Autodesk Fusion 360 part; units mm, degrees
note: some values were not read from the file. Set by a fixed rule: which sketch regions a step uses.
(part 2 of 3)
  line L917 (15.6798, -39.6054) -> (15.6321, -39.5578)
  line L918 (15.2055, -47.9863) -> (15.2532, -47.8435)
  line L919 (15.2532, -47.8435) -> (15.3008, -47.7959)
  line L920 (15.3008, -47.7959) -> (15.396, -47.7482)
  line L921 (15.396, -47.7482) -> (15.5389, -47.7482)
  line L922 (15.5389, -47.7482) -> (15.6341, -47.7959)
  line L923 (15.6341, -47.7959) -> (15.6817, -47.8435)
  line L924 (15.6817, -47.8435) -> (15.7293, -47.9387)
  line L925 (15.7293, -47.9387) -> (15.7293, -48.3197)
  line L926 (15.7293, -48.3197) -> (14.7293, -48.3197)
  line L927 (14.7293, -48.3197) -> (14.7293, -47.9863)
  line L928 (14.7293, -47.9863) -> (14.777, -47.8911)
  line L929 (14.777, -47.8911) -> (14.8246, -47.8435)
  line L930 (14.8246, -47.8435) -> (14.9198, -47.7959)
  line L931 (14.9198, -47.7959) -> (15.0151, -47.7959)
  line L932 (15.0151, -47.7959) -> (15.1103, -47.8435)
  line L933 (15.1103, -47.8435) -> (15.1579, -47.8911)
  line L934 (15.1579, -47.8911) -> (15.2055, -47.9863)
  line L935 (15.2055, -47.9863) -> (15.2055, -48.3197)
  line L936 (14.7293, -47.3197) -> (15.5389, -47.3197)
  line L937 (15.5389, -47.3197) -> (15.6341, -47.2721)
  line L938 (15.6341, -47.2721) -> (15.6817, -47.2244)
  line L939 (15.6817, -47.2244) -> (15.7293, -47.1292)
  line L940 (15.7293, -47.1292) -> (15.7293, -46.9387)
  line L941 (15.7293, -46.9387) -> (15.6817, -46.8435)
  line L942 (15.6817, -46.8435) -> (15.6341, -46.7959)
  line L943 (15.6341, -46.7959) -> (15.5389, -46.7482)
  line L944 (15.5389, -46.7482) -> (14.7293, -46.7482)
  line L945 (14.7293, -46.4149) -> (14.7293, -45.8435)
  line L946 (15.7293, -46.1292) -> (14.7293, -46.1292)
  line L947 (14.7293, -45.653) -> (14.7293, -45.0816)
  line L948 (15.7293, -45.3673) -> (14.7293, -45.3673)
  line L949 (14.7293, -44.5578) -> (14.7293, -44.3673)
  line L950 (14.7293, -44.3673) -> (14.777, -44.2721)
  line L951 (14.777, -44.2721) -> (14.8722, -44.1768)
  line L952 (14.8722, -44.1768) -> (15.0627, -44.1292)
  line L953 (15.0627, -44.1292) -> (15.396, -44.1292)
  line L954 (15.396, -44.1292) -> (15.5865, -44.1768)
  line L955 (15.5865, -44.1768) -> (15.6817, -44.2721)
  line L956 (15.6817, -44.2721) -> (15.7293, -44.3673)
  line L957 (15.7293, -44.3673) -> (15.7293, -44.5578)
  line L958 (15.7293, -44.5578) -> (15.6817, -44.653)
  line L959 (15.6817, -44.653) -> (15.5865, -44.7482)
  line L960 (15.5865, -44.7482) -> (15.396, -44.7959)
  line L961 (15.396, -44.7959) -> (15.0627, -44.7959)
  line L962 (15.0627, -44.7959) -> (14.8722, -44.7482)
  line L963 (14.8722, -44.7482) -> (14.777, -44.653)
  line L964 (14.777, -44.653) -> (14.7293, -44.5578)
  line L965 (15.7293, -43.7006) -> (14.7293, -43.7006)
  line L966 (14.7293, -43.7006) -> (15.7293, -43.1292)
  line L967 (15.7293, -43.1292) -> (14.7293, -43.1292)
  line L968 (15.6817, -42.7006) -> (15.7293, -42.5578)
  line L969 (15.7293, -42.5578) -> (15.7293, -42.3197)
  line L970 (15.7293, -42.3197) -> (15.6817, -42.2244)
  line L971 (15.6817, -42.2244) -> (15.6341, -42.1768)
  line L972 (15.6341, -42.1768) -> (15.5389, -42.1292)
  line L973 (15.5389, -42.1292) -> (15.4436, -42.1292)
  line L974 (15.4436, -42.1292) -> (15.3484, -42.1768)
  line L975 (15.3484, -42.1768) -> (15.3008, -42.2244)
  line L976 (15.3008, -42.2244) -> (15.2532, -42.3197)
  line L977 (15.2532, -42.3197) -> (15.2055, -42.5102)
  line L978 (15.2055, -42.5102) -> (15.1579, -42.6054)
  line L979 (15.1579, -42.6054) -> (15.1103, -42.653)
  line L980 (15.1103, -42.653) -> (15.0151, -42.7006)
  line L981 (15.0151, -42.7006) -> (14.9198, -42.7006)
  line L982 (14.9198, -42.7006) -> (14.8246, -42.653)
  line L983 (14.8246, -42.653) -> (14.777, -42.6054)
  line L984 (14.777, -42.6054) -> (14.7293, -42.5102)
  line L985 (14.7293, -42.5102) -> (14.7293, -42.2721)
  line L986 (14.7293, -42.2721) -> (14.777, -42.1292)
  line L987 (34.3226, -25.4531) -> (34.3226, -26.2626)
  line L988 (34.3226, -26.2626) -> (34.3702, -26.3578)
  line L989 (34.3702, -26.3578) -> (34.4179, -26.4054)
  line L990 (34.4179, -26.4054) -> (34.5131, -26.4531)
  line L991 (34.5131, -26.4531) -> (34.7036, -26.4531)
  line L992 (34.7036, -26.4531) -> (34.7988, -26.4054)
  line L993 (34.7988, -26.4054) -> (34.8464, -26.3578)
  line L994 (34.8464, -26.3578) -> (34.894, -26.2626)
  line L995 (34.894, -26.2626) -> (34.894, -25.4531)
  line L996 (35.894, -26.4531) -> (35.3226, -26.4531)
  line L997 (35.6083, -26.4531) -> (35.6083, -25.4531)
  line L998 (35.6083, -25.4531) -> (35.5131, -25.5959)
  line L999 (35.5131, -25.5959) -> (35.4179, -25.6912)
  line L1000 (35.4179, -25.6912) -> (35.3226, -25.7388)
  line L1001 (38.9893, -52.5224) -> (39.1036, -52.5605)
  line L1002 (39.1036, -52.5605) -> (39.294, -52.5605)
  line L1003 (39.294, -52.5605) -> (39.3702, -52.5224)
  line L1004 (39.3702, -52.5224) -> (39.4083, -52.4844)
  line L1005 (39.4083, -52.4844) -> (39.4464, -52.4082)
  line L1006 (39.4464, -52.4082) -> (39.4464, -52.332)
  line L1007 (39.4464, -52.332) -> (39.4083, -52.2558)
  line L1008 (39.4083, -52.2558) -> (39.3702, -52.2177)
  line L1009 (39.3702, -52.2177) -> (39.294, -52.1796)
  line L1010 (39.294, -52.1796) -> (39.1417, -52.1415)
  line L1011 (39.1417, -52.1415) -> (39.0655, -52.1034)
  line L1012 (39.0655, -52.1034) -> (39.0274, -52.0653)
  line L1013 (39.0274, -52.0653) -> (38.9893, -51.9891)
  line L1014 (38.9893, -51.9891) -> (38.9893, -51.9129)
  line L1015 (38.9893, -51.9129) -> (39.0274, -51.8367)
  line L1016 (39.0274, -51.8367) -> (39.0655, -51.7986)
  line L1017 (39.0655, -51.7986) -> (39.1417, -51.7605)
  line L1018 (39.1417, -51.7605) -> (39.3321, -51.7605)
  line L1019 (39.3321, -51.7605) -> (39.4464, -51.7986)
  line L1020 (39.7131, -51.7605) -> (39.9036, -52.5605)
  line L1021 (39.9036, -52.5605) -> (40.056, -51.9891)
  line L1022 (40.056, -51.9891) -> (40.2083, -52.5605)
  line L1023 (40.2083, -52.5605) -> (40.3988, -51.7605)
  line L1024 (40.7036, -52.5605) -> (40.7036, -51.7605)
  line L1025 (40.7036, -51.7605) -> (40.894, -51.7605)
  line L1026 (40.894, -51.7605) -> (41.0083, -51.7986)
  line L1027 (41.0083, -51.7986) -> (41.0845, -51.8748)
  line L1028 (41.0845, -51.8748) -> (41.1226, -51.951)
  line L1029 (41.1226, -51.951) -> (41.1607, -52.1034)
  line L1030 (41.1607, -52.1034) -> (41.1607, -52.2177)
  line L1031 (41.1607, -52.2177) -> (41.1226, -52.3701)
  line L1032 (41.1226, -52.3701) -> (41.0845, -52.4463)
  line L1033 (41.0845, -52.4463) -> (41.0083, -52.5224)
  line L1034 (41.0083, -52.5224) -> (40.894, -52.5605)
  line L1035 (40.894, -52.5605) -> (40.7036, -52.5605)
  line L1036 (41.5036, -52.5605) -> (41.5036, -51.7605)
  line L1037 (42.0369, -51.7605) -> (42.1893, -51.7605)
  line L1038 (42.1893, -51.7605) -> (42.2655, -51.7986)
  line L1039 (42.2655, -51.7986) -> (42.3417, -51.8748)
  line L1040 (42.3417, -51.8748) -> (42.3798, -52.0272)
  line L1041 (42.3798, -52.0272) -> (42.3798, -52.2939)
  line L1042 (42.3798, -52.2939) -> (42.3417, -52.4463)
  line L1043 (42.3417, -52.4463) -> (42.2655, -52.5224)
  line L1044 (42.2655, -52.5224) -> (42.1893, -52.5605)
  line L1045 (42.1893, -52.5605) -> (42.0369, -52.5605)
  line L1046 (42.0369, -52.5605) -> (41.9607, -52.5224)
  line L1047 (41.9607, -52.5224) -> (41.8845, -52.4463)
  line L1048 (41.8845, -52.4463) -> (41.8464, -52.2939)
  line L1049 (41.8464, -52.2939) -> (41.8464, -52.0272)
  line L1050 (41.8464, -52.0272) -> (41.8845, -51.8748)
  line L1051 (41.8845, -51.8748) -> (41.9607, -51.7986)
  line L1052 (41.9607, -51.7986) -> (42.0369, -51.7605)
  line L1053 (27.575, -52.5224) -> (27.6893, -52.5605)
  line L1054 (27.6893, -52.5605) -> (27.8798, -52.5605)
  line L1055 (27.8798, -52.5605) -> (27.956, -52.5224)
  line L1056 (27.956, -52.5224) -> (27.994, -52.4844)
  line L1057 (27.994, -52.4844) -> (28.0321, -52.4082)
  line L1058 (28.0321, -52.4082) -> (28.0321, -52.332)
  line L1059 (28.0321, -52.332) -> (27.994, -52.2558)
  line L1060 (27.994, -52.2558) -> (27.956, -52.2177)
  line L1061 (27.956, -52.2177) -> (27.8798, -52.1796)
  line L1062 (27.8798, -52.1796) -> (27.7274, -52.1415)
  line L1063 (27.7274, -52.1415) -> (27.6512, -52.1034)
  line L1064 (27.6512, -52.1034) -> (27.6131, -52.0653)
  line L1065 (27.6131, -52.0653) -> (27.575, -51.9891)
  line L1066 (27.575, -51.9891) -> (27.575, -51.9129)
  line L1067 (27.575, -51.9129) -> (27.6131, -51.8367)
  line L1068 (27.6131, -51.8367) -> (27.6512, -51.7986)
  line L1069 (27.6512, -51.7986) -> (27.7274, -51.7605)
  line L1070 (27.7274, -51.7605) -> (27.9179, -51.7605)
  line L1071 (27.9179, -51.7605) -> (28.0321, -51.7986)
  line L1072 (28.2988, -51.7605) -> (28.4893, -52.5605)
  line L1073 (28.4893, -52.5605) -> (28.6417, -51.9891)
  line L1074 (28.6417, -51.9891) -> (28.794, -52.5605)
  line L1075 (28.794, -52.5605) -> (28.9845, -51.7605)
  line L1076 (29.7464, -52.4844) -> (29.7083, -52.5224)
  line L1077 (29.7083, -52.5224) -> (29.594, -52.5605)
  line L1078 (29.594, -52.5605) -> (29.5179, -52.5605)
  line L1079 (29.5179, -52.5605) -> (29.4036, -52.5224)
  line L1080 (29.4036, -52.5224) -> (29.3274, -52.4463)
  line L1081 (29.3274, -52.4463) -> (29.2893, -52.3701)
  line L1082 (29.2893, -52.3701) -> (29.2512, -52.2177)
  line L1083 (29.2512, -52.2177) -> (29.2512, -52.1034)
  line L1084 (29.2512, -52.1034) -> (29.2893, -51.951)
  line L1085 (29.2893, -51.951) -> (29.3274, -51.8748)
  line L1086 (29.3274, -51.8748) -> (29.4036, -51.7986)
  line L1087 (29.4036, -51.7986) -> (29.5179, -51.7605)
  line L1088 (29.5179, -51.7605) -> (29.594, -51.7605)
  line L1089 (29.594, -51.7605) -> (29.7083, -51.7986)
  line L1090 (29.7083, -51.7986) -> (29.7464, -51.8367)
  line L1091 (30.4702, -52.5605) -> (30.0893, -52.5605)
  line L1092 (30.0893, -52.5605) -> (30.0893, -51.7605)
  line L1093 (30.7369, -52.5605) -> (30.7369, -51.7605)
  line L1094 (31.194, -52.5605) -> (30.8512, -52.1034)
  line L1095 (31.194, -51.7605) -> (30.7369, -52.2177)
  line L1096 (4.5155, -43.784) -> (4.5632, -43.6411)
  line L1097 (4.5632, -43.6411) -> (4.6108, -43.5935)
  line L1098 (4.6108, -43.5935) -> (4.706, -43.5459)
  line L1099 (4.706, -43.5459) -> (4.8489, -43.5459)
  line L1100 (4.8489, -43.5459) -> (4.9441, -43.5935)
  line L1101 (4.9441, -43.5935) -> (4.9917, -43.6411)
  line L1102 (4.9917, -43.6411) -> (5.0393, -43.7363)
  line L1103 (5.0393, -43.7363) -> (5.0393, -44.1173)
  line L1104 (5.0393, -44.1173) -> (4.0393, -44.1173)
  line L1105 (4.0393, -44.1173) -> (4.0393, -43.784)
  line L1106 (4.0393, -43.784) -> (4.087, -43.6887)
  line L1107 (4.087, -43.6887) -> (4.1346, -43.6411)
  line L1108 (4.1346, -43.6411) -> (4.2298, -43.5935)
  line L1109 (4.2298, -43.5935) -> (4.3251, -43.5935)
  line L1110 (4.3251, -43.5935) -> (4.4203, -43.6411)
  line L1111 (4.4203, -43.6411) -> (4.4679, -43.6887)
  line L1112 (4.4679, -43.6887) -> (4.5155, -43.784)
  line L1113 (4.5155, -43.784) -> (4.5155, -44.1173)
  line L1114 (4.0393, -43.2602) -> (4.0393, -42.6887)
  line L1115 (5.0393, -42.9744) -> (4.0393, -42.9744)
  line L1116 (5.0393, -41.8316) -> (5.0393, -42.403)
  line L1117 (5.0393, -42.1173) -> (4.0393, -42.1173)
  line L1118 (4.0393, -42.1173) -> (4.1822, -42.2125)
  line L1119 (4.1822, -42.2125) -> (4.2774, -42.3078)
  line L1120 (4.2774, -42.3078) -> (4.3251, -42.403)
  line L1121 (6.4441, -48.9506) -> (6.4917, -48.9982)
  line L1122 (6.4917, -48.9982) -> (6.5393, -49.1411)
  line L1123 (6.5393, -49.1411) -> (6.5393, -49.2363)
  line L1124 (6.5393, -49.2363) -> (6.4917, -49.3792)
  line L1125 (6.4917, -49.3792) -> (6.3965, -49.4744)
  line L1126 (6.3965, -49.4744) -> (6.3012, -49.5221)
  line L1127 (6.3012, -49.5221) -> (6.1108, -49.5697)
  line L1128 (6.1108, -49.5697) -> (5.9679, -49.5697)
  line L1129 (5.9679, -49.5697) -> (5.7774, -49.5221)
  line L1130 (5.7774, -49.5221) -> (5.6822, -49.4744)
  line L1131 (5.6822, -49.4744) -> (5.587, -49.3792)
  line L1132 (5.587, -49.3792) -> (5.5393, -49.2363)
  line L1133 (5.5393, -49.2363) -> (5.5393, -49.1411)
  line L1134 (5.5393, -49.1411) -> (5.587, -48.9982)
  line L1135 (5.587, -48.9982) -> (5.6346, -48.9506)
  line L1136 (6.5393, -47.9506) -> (6.0632, -48.284)
  line L1137 (6.5393, -48.5221) -> (5.5393, -48.5221)
  line L1138 (5.5393, -48.5221) -> (5.5393, -48.1411)
  line L1139 (5.5393, -48.1411) -> (5.587, -48.0459)
  line L1140 (5.587, -48.0459) -> (5.6346, -47.9982)
  line L1141 (5.6346, -47.9982) -> (5.7298, -47.9506)
  line L1142 (5.7298, -47.9506) -> (5.8727, -47.9506)
  line L1143 (5.8727, -47.9506) -> (5.9679, -47.9982)
  line L1144 (5.9679, -47.9982) -> (6.0155, -48.0459)
  line L1145 (6.0155, -48.0459) -> (6.0632, -48.1411)
  line L1146 (6.0632, -48.1411) -> (6.0632, -48.5221)
  line L1147 (5.6346, -47.5697) -> (5.587, -47.5221)
  line L1148 (5.587, -47.5221) -> (5.5393, -47.4268)
  line L1149 (5.5393, -47.4268) -> (5.5393, -47.1887)
  line L1150 (5.5393, -47.1887) -> (5.587, -47.0935)
  line L1151 (5.587, -47.0935) -> (5.6346, -47.0459)
  line L1152 (5.6346, -47.0459) -> (5.7298, -46.9982)
  line L1153 (5.7298, -46.9982) -> (5.8251, -46.9982)
  line L1154 (5.8251, -46.9982) -> (5.9679, -47.0459)
  line L1155 (5.9679, -47.0459) -> (6.5393, -47.6173)
  line L1156 (6.5393, -47.6173) -> (6.5393, -46.9982)
  line L1157 (5.5393, -46.3792) -> (5.5393, -46.284)
  line L1158 (5.5393, -46.284) -> (5.587, -46.1887)
  line L1159 (5.587, -46.1887) -> (5.6346, -46.1411)
  line L1160 (5.6346, -46.1411) -> (5.7298, -46.0935)
  line L1161 (5.7298, -46.0935) -> (5.9203, -46.0459)
  line L1162 (5.9203, -46.0459) -> (6.1584, -46.0459)
  line L1163 (6.1584, -46.0459) -> (6.3489, -46.0935)
  line L1164 (6.3489, -46.0935) -> (6.4441, -46.1411)
  line L1165 (6.4441, -46.1411) -> (6.4917, -46.1887)
  line L1166 (6.4917, -46.1887) -> (6.5393, -46.284)
  line L1167 (6.5393, -46.284) -> (6.5393, -46.3792)
  line L1168 (6.5393, -46.3792) -> (6.4917, -46.4744)
  line L1169 (6.4917, -46.4744) -> (6.4441, -46.5221)
  line L1170 (6.4441, -46.5221) -> (6.3489, -46.5697)
  line L1171 (6.3489, -46.5697) -> (6.1584, -46.6173)
  line L1172 (6.1584, -46.6173) -> (5.9203, -46.6173)
  line L1173 (5.9203, -46.6173) -> (5.7298, -46.5697)
  line L1174 (5.7298, -46.5697) -> (5.6346, -46.5221)
  line L1175 (5.6346, -46.5221) -> (5.587, -46.4744)
  line L1176 (5.587, -46.4744) -> (5.5393, -46.3792)
  line L1177 (5.5393, -45.7125) -> (5.5393, -45.0935)
  line L1178 (5.5393, -45.0935) -> (5.9203, -45.4268)
  line L1179 (5.9203, -45.4268) -> (5.9203, -45.284)
  line L1180 (5.9203, -45.284) -> (5.9679, -45.1887)
  line L1181 (5.9679, -45.1887) -> (6.0155, -45.1411)
  line L1182 (6.0155, -45.1411) -> (6.1108, -45.0935)
  line L1183 (6.1108, -45.0935) -> (6.3489, -45.0935)
  line L1184 (6.3489, -45.0935) -> (6.4441, -45.1411)
  line L1185 (6.4441, -45.1411) -> (6.4917, -45.1887)
  line L1186 (6.4917, -45.1887) -> (6.5393, -45.284)
  line L1187 (6.5393, -45.284) -> (6.5393, -45.5697)
  line L1188 (6.5393, -45.5697) -> (6.4917, -45.6649)
  line L1189 (6.4917, -45.6649) -> (6.4441, -45.7125)
  line L1190 (5.6346, -44.7125) -> (5.587, -44.6649)
  line L1191 (5.587, -44.6649) -> (5.5393, -44.5697)
  line L1192 (5.5393, -44.5697) -> (5.5393, -44.3316)
  line L1193 (5.5393, -44.3316) -> (5.587, -44.2363)
  line L1194 (5.587, -44.2363) -> (5.6346, -44.1887)
  line L1195 (5.6346, -44.1887) -> (5.7298, -44.1411)
  line L1196 (5.7298, -44.1411) -> (5.8251, -44.1411)
  line L1197 (5.8251, -44.1411) -> (5.9679, -44.1887)
  line L1198 (5.9679, -44.1887) -> (6.5393, -44.7602)
  line L1199 (6.5393, -44.7602) -> (6.5393, -44.1411)
  line L1200 (6.6346, -43.9506) -> (6.6346, -43.1887)
  line L1201 (6.4441, -42.3792) -> (6.4917, -42.4268)
  line L1202 (6.4917, -42.4268) -> (6.5393, -42.5697)
  line L1203 (6.5393, -42.5697) -> (6.5393, -42.6649)
  line L1204 (6.5393, -42.6649) -> (6.4917, -42.8078)
  line L1205 (6.4917, -42.8078) -> (6.3965, -42.903)
  line L1206 (6.3965, -42.903) -> (6.3012, -42.9506)
  line L1207 (6.3012, -42.9506) -> (6.1108, -42.9982)
  line L1208 (6.1108, -42.9982) -> (5.9679, -42.9982)
  line L1209 (5.9679, -42.9982) -> (5.7774, -42.9506)
  line L1210 (5.7774, -42.9506) -> (5.6822, -42.903)
  line L1211 (5.6822, -42.903) -> (5.587, -42.8078)
  line L1212 (5.587, -42.8078) -> (5.5393, -42.6649)
  line L1213 (5.5393, -42.6649) -> (5.5393, -42.5697)
  line L1214 (5.5393, -42.5697) -> (5.587, -42.4268)
  line L1215 (5.587, -42.4268) -> (5.6346, -42.3792)
  line L1216 (6.5393, -41.8078) -> (6.4917, -41.903)
  line L1217 (6.4917, -41.903) -> (6.4441, -41.9506)
  line L1218 (6.4441, -41.9506) -> (6.3489, -41.9982)
  line L1219 (6.3489, -41.9982) -> (6.0632, -41.9982)
  line L1220 (6.0632, -41.9982) -> (5.9679, -41.9506)
  line L1221 (5.9679, -41.9506) -> (5.9203, -41.903)
  line L1222 (5.9203, -41.903) -> (5.8727, -41.8078)
  line L1223 (5.8727, -41.8078) -> (5.8727, -41.6649)
  line L1224 (5.8727, -41.6649) -> (5.9203, -41.5697)
  line L1225 (5.9203, -41.5697) -> (5.9679, -41.5221)
  line L1226 (5.9679, -41.5221) -> (6.0632, -41.4744)
  line L1227 (6.0632, -41.4744) -> (6.3489, -41.4744)
  line L1228 (6.3489, -41.4744) -> (6.4441, -41.5221)
  line L1229 (6.4441, -41.5221) -> (6.4917, -41.5697)
  line L1230 (6.4917, -41.5697) -> (6.5393, -41.6649)
  line L1231 (6.5393, -41.6649) -> (6.5393, -41.8078)
  line L1232 (6.5393, -41.0459) -> (5.8727, -41.0459)
  line L1233 (5.5393, -41.0459) -> (5.587, -41.0935)
  line L1234 (5.587, -41.0935) -> (5.6346, -41.0459)
  line L1235 (5.6346, -41.0459) -> (5.587, -40.9982)
  line L1236 (5.587, -40.9982) -> (5.5393, -41.0459)
  line L1237 (5.5393, -41.0459) -> (5.6346, -41.0459)
  line L1238 (5.8727, -40.5697) -> (6.5393, -40.5697)
  line L1239 (5.9679, -40.5697) -> (5.9203, -40.5221)
  line L1240 (5.9203, -40.5221) -> (5.8727, -40.4268)
  line L1241 (5.8727, -40.4268) -> (5.8727, -40.284)
  line L1242 (5.8727, -40.284) -> (5.9203, -40.1887)
  line L1243 (5.9203, -40.1887) -> (6.0155, -40.1411)
  line L1244 (6.0155, -40.1411) -> (6.5393, -40.1411)
  line L1245 (6.6346, -39.903) -> (6.6346, -39.1411)
  line L1246 (6.4441, -38.3316) -> (6.4917, -38.3792)
  line L1247 (6.4917, -38.3792) -> (6.5393, -38.5221)
  line L1248 (6.5393, -38.5221) -> (6.5393, -38.6173)
  line L1249 (6.5393, -38.6173) -> (6.4917, -38.7602)
  line L1250 (6.4917, -38.7602) -> (6.3965, -38.8554)
  line L1251 (6.3965, -38.8554) -> (6.3012, -38.903)
  line L1252 (6.3012, -38.903) -> (6.1108, -38.9506)
  line L1253 (6.1108, -38.9506) -> (5.9679, -38.9506)
  line L1254 (5.9679, -38.9506) -> (5.7774, -38.903)
  line L1255 (5.7774, -38.903) -> (5.6822, -38.8554)
  line L1256 (5.6822, -38.8554) -> (5.587, -38.7602)
  line L1257 (5.587, -38.7602) -> (5.5393, -38.6173)
  line L1258 (5.5393, -38.6173) -> (5.5393, -38.5221)
  line L1259 (5.5393, -38.5221) -> (5.587, -38.3792)
  line L1260 (5.587, -38.3792) -> (5.6346, -38.3316)
  line L1261 (6.4917, -37.5221) -> (6.5393, -37.6173)
  line L1262 (6.5393, -37.6173) -> (6.5393, -37.8078)
  line L1263 (6.5393, -37.8078) -> (6.4917, -37.903)
  line L1264 (6.4917, -37.903) -> (6.3965, -37.9506)
  line L1265 (6.3965, -37.9506) -> (6.0155, -37.9506)
  line L1266 (6.0155, -37.9506) -> (5.9203, -37.903)
  line L1267 (5.9203, -37.903) -> (5.8727, -37.8078)
  line L1268 (5.8727, -37.8078) -> (5.8727, -37.6173)
  line L1269 (5.8727, -37.6173) -> (5.9203, -37.5221)
  line L1270 (5.9203, -37.5221) -> (6.0155, -37.4744)
  line L1271 (6.0155, -37.4744) -> (6.1108, -37.4744)
  line L1272 (6.1108, -37.4744) -> (6.206, -37.9506)
  line L1273 (6.5393, -36.903) -> (6.4917, -36.9982)
  line L1274 (6.4917, -36.9982) -> (6.3965, -37.0459)
  line L1275 (6.3965, -37.0459) -> (5.5393, -37.0459)
  line L1276 (6.5393, -36.3792) -> (6.4917, -36.4744)
  line L1277 (6.4917, -36.4744) -> (6.3965, -36.5221)
  line L1278 (6.3965, -36.5221) -> (5.5393, -36.5221)
  line L1279 (63.2012, -15.1656) -> (63.2012, -15.8799)
  line L1280 (63.2012, -15.8799) -> (63.1536, -16.0227)
  line L1281 (63.1536, -16.0227) -> (63.0583, -16.118)
  line L1282 (63.0583, -16.118) -> (62.9155, -16.1656)
  line L1283 (62.9155, -16.1656) -> (62.8202, -16.1656)
  line L1284 (64.1536, -15.1656) -> (63.6774, -15.1656)
  line L1285 (63.6774, -15.1656) -> (63.6298, -15.6418)
  line L1286 (63.6298, -15.6418) -> (63.6774, -15.5941)
  line L1287 (63.6774, -15.5941) -> (63.7726, -15.5465)
  line L1288 (63.7726, -15.5465) -> (64.0107, -15.5465)
  line L1289 (64.0107, -15.5465) -> (64.106, -15.5941)
  line L1290 (64.106, -15.5941) -> (64.1536, -15.6418)
  line L1291 (64.1536, -15.6418) -> (64.2012, -15.737)
  line L1292 (64.2012, -15.737) -> (64.2012, -15.9751)
  line L1293 (64.2012, -15.9751) -> (64.1536, -16.0703)
  line L1294 (64.1536, -16.0703) -> (64.106, -16.118)
  line L1295 (64.106, -16.118) -> (64.0107, -16.1656)
  line L1296 (64.0107, -16.1656) -> (63.7726, -16.1656)
  line L1297 (63.7726, -16.1656) -> (63.6774, -16.118)
  line L1298 (63.6774, -16.118) -> (63.6298, -16.0703)
  line L1299 (66.0393, -6.9863) -> (66.8489, -6.9863)
  line L1300 (66.8489, -6.9863) -> (66.9441, -6.9387)
  line L1301 (66.9441, -6.9387) -> (66.9917, -6.8911)
  line L1302 (66.9917, -6.8911) -> (67.0393, -6.7959)
  line L1303 (67.0393, -6.7959) -> (67.0393, -6.6054)
  line L1304 (67.0393, -6.6054) -> (66.9917, -6.5102)
  line L1305 (66.9917, -6.5102) -> (66.9441, -6.4625)
  line L1306 (66.9441, -6.4625) -> (66.8489, -6.4149)
  line L1307 (66.8489, -6.4149) -> (66.0393, -6.4149)
  line L1308 (66.9917, -5.9863) -> (67.0393, -5.8435)
  line L1309 (67.0393, -5.8435) -> (67.0393, -5.6054)
  line L1310 (67.0393, -5.6054) -> (66.9917, -5.5102)
  line L1311 (66.9917, -5.5102) -> (66.9441, -5.4625)
  line L1312 (66.9441, -5.4625) -> (66.8489, -5.4149)
  line L1313 (66.8489, -5.4149) -> (66.7536, -5.4149)
  line L1314 (66.7536, -5.4149) -> (66.6584, -5.4625)
  line L1315 (66.6584, -5.4625) -> (66.6108, -5.5102)
  line L1316 (66.6108, -5.5102) -> (66.5632, -5.6054)
  line L1317 (66.5632, -5.6054) -> (66.5155, -5.7959)
  line L1318 (66.5155, -5.7959) -> (66.4679, -5.8911)
  line L1319 (66.4679, -5.8911) -> (66.4203, -5.9387)
  line L1320 (66.4203, -5.9387) -> (66.3251, -5.9863)
  line L1321 (66.3251, -5.9863) -> (66.2298, -5.9863)
  line L1322 (66.2298, -5.9863) -> (66.1346, -5.9387)
  line L1323 (66.1346, -5.9387) -> (66.087, -5.8911)
  line L1324 (66.087, -5.8911) -> (66.0393, -5.7959)
  line L1325 (66.0393, -5.7959) -> (66.0393, -5.5578)
  line L1326 (66.0393, -5.5578) -> (66.087, -5.4149)
  line L1327 (66.5155, -4.653) -> (66.5632, -4.5102)
  line L1328 (66.5632, -4.5102) -> (66.6108, -4.4625)
  line L1329 (66.6108, -4.4625) -> (66.706, -4.4149)
  line L1330 (66.706, -4.4149) -> (66.8489, -4.4149)
  line L1331 (66.8489, -4.4149) -> (66.9441, -4.4625)
  line L1332 (66.9441, -4.4625) -> (66.9917, -4.5102)
  line L1333 (66.9917, -4.5102) -> (67.0393, -4.6054)
  line L1334 (67.0393, -4.6054) -> (67.0393, -4.9863)
  line L1335 (67.0393, -4.9863) -> (66.0393, -4.9863)
  line L1336 (66.0393, -4.9863) -> (66.0393, -4.653)
  line L1337 (66.0393, -4.653) -> (66.087, -4.5578)
  line L1338 (66.087, -4.5578) -> (66.1346, -4.5102)
  line L1339 (66.1346, -4.5102) -> (66.2298, -4.4625)
  line L1340 (66.2298, -4.4625) -> (66.3251, -4.4625)
  line L1341 (66.3251, -4.4625) -> (66.4203, -4.5102)
  line L1342 (66.4203, -4.5102) -> (66.4679, -4.5578)
  line L1343 (66.4679, -4.5578) -> (66.5155, -4.653)
  line L1344 (66.5155, -4.653) -> (66.5155, -4.9863)
  line L1345 (66.1346, -4.034) -> (66.087, -3.9863)
  line L1346 (66.087, -3.9863) -> (66.0393, -3.8911)
  line L1347 (66.0393, -3.8911) -> (66.0393, -3.653)
  line L1348 (66.0393, -3.653) -> (66.087, -3.5578)
  line L1349 (66.087, -3.5578) -> (66.1346, -3.5102)
  line L1350 (66.1346, -3.5102) -> (66.2298, -3.4625)
  line L1351 (66.2298, -3.4625) -> (66.3251, -3.4625)
  line L1352 (66.3251, -3.4625) -> (66.4679, -3.5102)
  line L1353 (66.4679, -3.5102) -> (67.0393, -4.0816)
  line L1354 (67.0393, -4.0816) -> (67.0393, -3.4625)
  line L1355 (5.9893, -21.5483) -> (5.894, -21.5007)
  line L1356 (5.894, -21.5007) -> (5.7988, -21.4055)
  line L1357 (5.7988, -21.4055) -> (5.656, -21.2626)
  line L1358 (5.656, -21.2626) -> (5.5607, -21.215)
  line L1359 (5.5607, -21.215) -> (5.4655, -21.215)
  line L1360 (5.5131, -21.4531) -> (5.4179, -21.4055)
  line L1361 (5.4179, -21.4055) -> (5.3226, -21.3102)
  line L1362 (5.3226, -21.3102) -> (5.275, -21.1197)
  line L1363 (5.275, -21.1197) -> (5.275, -20.7864)
  line L1364 (5.275, -20.7864) -> (5.3226, -20.5959)
  line L1365 (5.3226, -20.5959) -> (5.4179, -20.5007)
  line L1366 (5.4179, -20.5007) -> (5.5131, -20.4531)
  line L1367 (5.5131, -20.4531) -> (5.7036, -20.4531)
  line L1368 (5.7036, -20.4531) -> (5.7988, -20.5007)
  line L1369 (5.7988, -20.5007) -> (5.894, -20.5959)
  line L1370 (5.894, -20.5959) -> (5.9417, -20.7864)
  line L1371 (5.9417, -20.7864) -> (5.9417, -21.1197)
  line L1372 (5.9417, -21.1197) -> (5.894, -21.3102)
  line L1373 (5.894, -21.3102) -> (5.7988, -21.4055)
  line L1374 (5.7988, -21.4055) -> (5.7036, -21.4531)
  line L1375 (5.7036, -21.4531) -> (5.5131, -21.4531)
  line L1376 (6.894, -21.4531) -> (6.3226, -21.4531)
  line L1377 (6.6083, -21.4531) -> (6.6083, -20.4531)
  line L1378 (6.6083, -20.4531) -> (6.5131, -20.5959)
  line L1379 (6.5131, -20.5959) -> (6.4179, -20.6912)
  line L1380 (6.4179, -20.6912) -> (6.3226, -20.7388)
  line L1381 (2.1346, -19.9625) -> (2.087, -19.9149)
  line L1382 (2.087, -19.9149) -> (2.0393, -19.8197)
  line L1383 (2.0393, -19.8197) -> (2.0393, -19.5816)
  line L1384 (2.0393, -19.5816) -> (2.087, -19.4863)
  line L1385 (2.087, -19.4863) -> (2.1346, -19.4387)
  line L1386 (2.1346, -19.4387) -> (2.2298, -19.3911)
  line L1387 (2.2298, -19.3911) -> (2.3251, -19.3911)
  line L1388 (2.3251, -19.3911) -> (2.4679, -19.4387)
  line L1389 (2.4679, -19.4387) -> (3.0393, -20.0102)
  line L1390 (3.0393, -20.0102) -> (3.0393, -19.3911)
  line L1391 (3.0393, -18.9625) -> (2.0393, -18.9625)
  line L1392 (2.0393, -18.9625) -> (3.0393, -18.3911)
  line L1393 (3.0393, -18.3911) -> (2.0393, -18.3911)
  line L1394 (2.0393, -18.0102) -> (2.0393, -17.3911)
  line L1395 (2.0393, -17.3911) -> (2.4203, -17.7244)
  line L1396 (2.4203, -17.7244) -> (2.4203, -17.5816)
  line L1397 (2.4203, -17.5816) -> (2.4679, -17.4863)
  line L1398 (2.4679, -17.4863) -> (2.5155, -17.4387)
  line L1399 (2.5155, -17.4387) -> (2.6108, -17.3911)
  line L1400 (2.6108, -17.3911) -> (2.8489, -17.3911)
  line L1401 (2.8489, -17.3911) -> (2.9441, -17.4387)
  line L1402 (2.9441, -17.4387) -> (2.9917, -17.4863)
  line L1403 (2.9917, -17.4863) -> (3.0393, -17.5816)
  line L1404 (3.0393, -17.5816) -> (3.0393, -17.8673)
  line L1405 (3.0393, -17.8673) -> (2.9917, -17.9625)
  line L1406 (2.9917, -17.9625) -> (2.9441, -18.0102)
  line L1407 (3.0393, -16.9149) -> (3.0393, -16.7244)
  line L1408 (3.0393, -16.7244) -> (2.9917, -16.6292)
  line L1409 (2.9917, -16.6292) -> (2.9441, -16.5816)
  line L1410 (2.9441, -16.5816) -> (2.8012, -16.4863)
  line L1411 (2.8012, -16.4863) -> (2.6108, -16.4387)
  line L1412 (2.6108, -16.4387) -> (2.2298, -16.4387)
  line L1413 (2.2298, -16.4387) -> (2.1346, -16.4863)
  line L1414 (2.1346, -16.4863) -> (2.087, -16.534)
  line L1415 (2.087, -16.534) -> (2.0393, -16.6292)
  line L1416 (2.0393, -16.6292) -> (2.0393, -16.8197)
  line L1417 (2.0393, -16.8197) -> (2.087, -16.9149)
  line L1418 (2.087, -16.9149) -> (2.1346, -16.9625)
  line L1419 (2.1346, -16.9625) -> (2.2298, -17.0102)
  line L1420 (2.2298, -17.0102) -> (2.4679, -17.0102)
  line L1421 (2.4679, -17.0102) -> (2.5632, -16.9625)
  line L1422 (2.5632, -16.9625) -> (2.6108, -16.9149)
  line L1423 (2.6108, -16.9149) -> (2.6584, -16.8197)
  line L1424 (2.6584, -16.8197) -> (2.6584, -16.6292)
  line L1425 (2.6584, -16.6292) -> (2.6108, -16.534)
  line L1426 (2.6108, -16.534) -> (2.5632, -16.4863)
  line L1427 (2.5632, -16.4863) -> (2.4679, -16.4387)
  line L1428 (2.0393, -15.8197) -> (2.0393, -15.7244)
  line L1429 (2.0393, -15.7244) -> (2.087, -15.6292)
  line L1430 (2.087, -15.6292) -> (2.1346, -15.5816)
  line L1431 (2.1346, -15.5816) -> (2.2298, -15.534)
  line L1432 (2.2298, -15.534) -> (2.4203, -15.4863)
  line L1433 (2.4203, -15.4863) -> (2.6584, -15.4863)
  line L1434 (2.6584, -15.4863) -> (2.8489, -15.534)
  line L1435 (2.8489, -15.534) -> (2.9441, -15.5816)
  line L1436 (2.9441, -15.5816) -> (2.9917, -15.6292)
  line L1437 (2.9917, -15.6292) -> (3.0393, -15.7244)
  line L1438 (3.0393, -15.7244) -> (3.0393, -15.8197)
  line L1439 (3.0393, -15.8197) -> (2.9917, -15.9149)
  line L1440 (2.9917, -15.9149) -> (2.9441, -15.9625)
  line L1441 (2.9441, -15.9625) -> (2.8489, -16.0102)
  line L1442 (2.8489, -16.0102) -> (2.6584, -16.0578)
  line L1443 (2.6584, -16.0578) -> (2.4203, -16.0578)
  line L1444 (2.4203, -16.0578) -> (2.2298, -16.0102)
  line L1445 (2.2298, -16.0102) -> (2.1346, -15.9625)
  line L1446 (2.1346, -15.9625) -> (2.087, -15.9149)
  line L1447 (2.087, -15.9149) -> (2.0393, -15.8197)
  line L1448 (2.3727, -14.6292) -> (3.0393, -14.6292)
  line L1449 (1.9917, -14.8673) -> (2.706, -15.1054)
  line L1450 (2.706, -15.1054) -> (2.706, -14.4863)
  line L1451 (15.2512, -29.8531) -> (15.2512, -30.5674)
  line L1452 (15.2512, -30.5674) -> (15.2036, -30.7102)
  line L1453 (15.2036, -30.7102) -> (15.1083, -30.8055)
  line L1454 (15.1083, -30.8055) -> (14.9655, -30.8531)
  line L1455 (14.9655, -30.8531) -> (14.8702, -30.8531)
  line L1456 (16.2512, -30.8531) -> (15.6798, -30.8531)
  line L1457 (15.9655, -30.8531) -> (15.9655, -29.8531)
  line L1458 (15.9655, -29.8531) -> (15.8702, -29.9959)
  line L1459 (15.8702, -29.9959) -> (15.775, -30.0912)
  line L1460 (15.775, -30.0912) -> (15.6798, -30.1388)
  line L1461 (15.7293, -35.3466) -> (15.7293, -35.8228)
  line L1462 (15.7293, -35.8228) -> (14.7293, -35.8228)
  line L1463 (15.7293, -35.0132) -> (14.7293, -35.0132)
  line L1464 (14.777, -34.0132) -> (14.7293, -34.1085)
  line L1465 (14.7293, -34.1085) -> (14.7293, -34.2513)
  line L1466 (14.7293, -34.2513) -> (14.777, -34.3942)
  line L1467 (14.777, -34.3942) -> (14.8722, -34.4894)
  line L1468 (14.8722, -34.4894) -> (14.9674, -34.5371)
  line L1469 (14.9674, -34.5371) -> (15.1579, -34.5847)
  line L1470 (15.1579, -34.5847) -> (15.3008, -34.5847)
  line L1471 (15.3008, -34.5847) -> (15.4912, -34.5371)
  line L1472 (15.4912, -34.5371) -> (15.5865, -34.4894)
  line L1473 (15.5865, -34.4894) -> (15.6817, -34.3942)
  line L1474 (15.6817, -34.3942) -> (15.7293, -34.2513)
  line L1475 (15.7293, -34.2513) -> (15.7293, -34.1561)
  line L1476 (15.7293, -34.1561) -> (15.6817, -34.0132)
  line L1477 (15.6817, -34.0132) -> (15.6341, -33.9656)
  line L1478 (15.6341, -33.9656) -> (15.3008, -33.9656)
  line L1479 (15.3008, -33.9656) -> (15.3008, -34.1561)
  line L1480 (15.7293, -33.5371) -> (14.7293, -33.5371)
  line L1481 (15.2055, -33.5371) -> (15.2055, -32.9656)
  line L1482 (15.7293, -32.9656) -> (14.7293, -32.9656)
  line L1483 (14.7293, -32.6323) -> (14.7293, -32.0609)
  line L1484 (15.7293, -32.3466) -> (14.7293, -32.3466)
  line L1485 (51.7712, -32.1706) -> (51.7712, -32.8849)
  line L1486 (51.7712, -32.8849) -> (51.7236, -33.0277)
  line L1487 (51.7236, -33.0277) -> (51.6283, -33.1229)
  line L1488 (51.6283, -33.1229) -> (51.4855, -33.1706)
  line L1489 (51.4855, -33.1706) -> (51.3902, -33.1706)
  line L1490 (52.1998, -32.2658) -> (52.2474, -32.2182)
  line L1491 (52.2474, -32.2182) -> (52.3426, -32.1706)
  line L1492 (52.3426, -32.1706) -> (52.5807, -32.1706)
  line L1493 (52.5807, -32.1706) -> (52.676, -32.2182)
  line L1494 (52.676, -32.2182) -> (52.7236, -32.2658)
  line L1495 (52.7236, -32.2658) -> (52.7712, -32.361)
  line L1496 (52.7712, -32.361) -> (52.7712, -32.4563)
  line L1497 (52.7712, -32.4563) -> (52.7236, -32.5991)
  line L1498 (52.7236, -32.5991) -> (52.1521, -33.1706)
  line L1499 (52.1521, -33.1706) -> (52.7712, -33.1706)
  line L1500 (54.0993, -44.1231) -> (54.0993, -43.9327)
  line L1501 (54.0993, -43.9327) -> (54.147, -43.8374)
  line L1502 (54.147, -43.8374) -> (54.2422, -43.7422)
  line L1503 (54.2422, -43.7422) -> (54.4327, -43.6946)
  line L1504 (54.4327, -43.6946) -> (54.766, -43.6946)
  line L1505 (54.766, -43.6946) -> (54.9565, -43.7422)
  line L1506 (54.9565, -43.7422) -> (55.0517, -43.8374)
  line L1507 (55.0517, -43.8374) -> (55.0993, -43.9327)
  line L1508 (55.0993, -43.9327) -> (55.0993, -44.1231)
  line L1509 (55.0993, -44.1231) -> (55.0517, -44.2184)
  line L1510 (55.0517, -44.2184) -> (54.9565, -44.3136)
  line L1511 (54.9565, -44.3136) -> (54.766, -44.3612)
  line L1512 (54.766, -44.3612) -> (54.4327, -44.3612)
  line L1513 (54.4327, -44.3612) -> (54.2422, -44.3136)
  line L1514 (54.2422, -44.3136) -> (54.147, -44.2184)
  line L1515 (54.147, -44.2184) -> (54.0993, -44.1231)
  line L1516 (55.0993, -42.7898) -> (55.0993, -43.266)
  line L1517 (55.0993, -43.266) -> (54.0993, -43.266)
  line L1518 (54.5755, -42.4565) -> (54.5755, -42.1231)
  line L1519 (55.0993, -41.9803) -> (55.0993, -42.4565)
  line L1520 (55.0993, -42.4565) -> (54.0993, -42.4565)
  line L1521 (54.0993, -42.4565) -> (54.0993, -41.9803)
  line L1522 (55.0993, -41.5517) -> (54.0993, -41.5517)
  line L1523 (54.0993, -41.5517) -> (54.0993, -41.3136)
  line L1524 (54.0993, -41.3136) -> (54.147, -41.1707)
  line L1525 (54.147, -41.1707) -> (54.2422, -41.0755)
  line L1526 (54.2422, -41.0755) -> (54.3374, -41.0279)
  line L1527 (54.3374, -41.0279) -> (54.5279, -40.9803)
  line L1528 (54.5279, -40.9803) -> (54.6708, -40.9803)
  line L1529 (54.6708, -40.9803) -> (54.8612, -41.0279)
  line L1530 (54.8612, -41.0279) -> (54.9565, -41.0755)
  line L1531 (54.9565, -41.0755) -> (55.0517, -41.1707)
  line L1532 (55.0517, -41.1707) -> (55.0993, -41.3136)
  line L1533 (55.0993, -41.3136) -> (55.0993, -41.5517)
  line L1534 (51.9893, -22.0483) -> (51.894, -22.0007)
  line L1535 (51.894, -22.0007) -> (51.7988, -21.9055)
  line L1536 (51.7988, -21.9055) -> (51.656, -21.7626)
  line L1537 (51.656, -21.7626) -> (51.5607, -21.715)
  line L1538 (51.5607, -21.715) -> (51.4655, -21.715)
  line L1539 (51.5131, -21.9531) -> (51.4179, -21.9055)
  line L1540 (51.4179, -21.9055) -> (51.3226, -21.8102)
  line L1541 (51.3226, -21.8102) -> (51.275, -21.6197)
  line L1542 (51.275, -21.6197) -> (51.275, -21.2864)
  line L1543 (51.275, -21.2864) -> (51.3226, -21.0959)
  line L1544 (51.3226, -21.0959) -> (51.4179, -21.0007)
  line L1545 (51.4179, -21.0007) -> (51.5131, -20.9531)
  line L1546 (51.5131, -20.9531) -> (51.7036, -20.9531)
  line L1547 (51.7036, -20.9531) -> (51.7988, -21.0007)
  line L1548 (51.7988, -21.0007) -> (51.894, -21.0959)
  line L1549 (51.894, -21.0959) -> (51.9417, -21.2864)
  line L1550 (51.9417, -21.2864) -> (51.9417, -21.6197)
  line L1551 (51.9417, -21.6197) -> (51.894, -21.8102)
  line L1552 (51.894, -21.8102) -> (51.7988, -21.9055)
  line L1553 (51.7988, -21.9055) -> (51.7036, -21.9531)
  line L1554 (51.7036, -21.9531) -> (51.5131, -21.9531)
  line L1555 (52.3226, -21.0483) -> (52.3702, -21.0007)
  line L1556 (52.3702, -21.0007) -> (52.4655, -20.9531)
  line L1557 (52.4655, -20.9531) -> (52.7036, -20.9531)
  line L1558 (52.7036, -20.9531) -> (52.7988, -21.0007)
  line L1559 (52.7988, -21.0007) -> (52.8464, -21.0483)
  line L1560 (52.8464, -21.0483) -> (52.894, -21.1435)
  line L1561 (52.894, -21.1435) -> (52.894, -21.2388)
  line L1562 (52.894, -21.2388) -> (52.8464, -21.3816)
  line L1563 (52.8464, -21.3816) -> (52.275, -21.9531)
  line L1564 (52.275, -21.9531) -> (52.894, -21.9531)
  line L1565 (55.6346, -20.4625) -> (55.587, -20.4149)
  line L1566 (55.587, -20.4149) -> (55.5393, -20.3197)
  line L1567 (55.5393, -20.3197) -> (55.5393, -20.0816)
  line L1568 (55.5393, -20.0816) -> (55.587, -19.9863)
  line L1569 (55.587, -19.9863) -> (55.6346, -19.9387)
  line L1570 (55.6346, -19.9387) -> (55.7298, -19.8911)
  line L1571 (55.7298, -19.8911) -> (55.8251, -19.8911)
  line L1572 (55.8251, -19.8911) -> (55.9679, -19.9387)
  line L1573 (55.9679, -19.9387) -> (56.5393, -20.5102)
  line L1574 (56.5393, -20.5102) -> (56.5393, -19.8911)
  line L1575 (56.5393, -19.4625) -> (55.5393, -19.4625)
  line L1576 (55.5393, -19.4625) -> (56.5393, -18.8911)
  line L1577 (56.5393, -18.8911) -> (55.5393, -18.8911)
  line L1578 (55.5393, -18.5102) -> (55.5393, -17.8911)
  line L1579 (55.5393, -17.8911) -> (55.9203, -18.2244)
  line L1580 (55.9203, -18.2244) -> (55.9203, -18.0816)
  line L1581 (55.9203, -18.0816) -> (55.9679, -17.9863)
  line L1582 (55.9679, -17.9863) -> (56.0155, -17.9387)
  line L1583 (56.0155, -17.9387) -> (56.1108, -17.8911)
  line L1584 (56.1108, -17.8911) -> (56.3489, -17.8911)
  line L1585 (56.3489, -17.8911) -> (56.4441, -17.9387)
  line L1586 (56.4441, -17.9387) -> (56.4917, -17.9863)
  line L1587 (56.4917, -17.9863) -> (56.5393, -18.0816)
  line L1588 (56.5393, -18.0816) -> (56.5393, -18.3673)
  line L1589 (56.5393, -18.3673) -> (56.4917, -18.4625)
  line L1590 (56.4917, -18.4625) -> (56.4441, -18.5102)
  line L1591 (56.5393, -17.4149) -> (56.5393, -17.2244)
  line L1592 (56.5393, -17.2244) -> (56.4917, -17.1292)
  line L1593 (56.4917, -17.1292) -> (56.4441, -17.0816)
  line L1594 (56.4441, -17.0816) -> (56.3012, -16.9863)
  line L1595 (56.3012, -16.9863) -> (56.1108, -16.9387)
  line L1596 (56.1108, -16.9387) -> (55.7298, -16.9387)
  line L1597 (55.7298, -16.9387) -> (55.6346, -16.9863)
  line L1598 (55.6346, -16.9863) -> (55.587, -17.034)
  line L1599 (55.587, -17.034) -> (55.5393, -17.1292)
  line L1600 (55.5393, -17.1292) -> (55.5393, -17.3197)
  line L1601 (55.5393, -17.3197) -> (55.587, -17.4149)
  line L1602 (55.587, -17.4149) -> (55.6346, -17.4625)
  line L1603 (55.6346, -17.4625) -> (55.7298, -17.5102)
  line L1604 (55.7298, -17.5102) -> (55.9679, -17.5102)
  line L1605 (55.9679, -17.5102) -> (56.0632, -17.4625)
  line L1606 (56.0632, -17.4625) -> (56.1108, -17.4149)
  line L1607 (56.1108, -17.4149) -> (56.1584, -17.3197)
  line L1608 (56.1584, -17.3197) -> (56.1584, -17.1292)
  line L1609 (56.1584, -17.1292) -> (56.1108, -17.034)
  line L1610 (56.1108, -17.034) -> (56.0632, -16.9863)
  line L1611 (56.0632, -16.9863) -> (55.9679, -16.9387)
  line L1612 (55.5393, -16.3197) -> (55.5393, -16.2244)
  line L1613 (55.5393, -16.2244) -> (55.587, -16.1292)
  line L1614 (55.587, -16.1292) -> (55.6346, -16.0816)
  line L1615 (55.6346, -16.0816) -> (55.7298, -16.034)
  line L1616 (55.7298, -16.034) -> (55.9203, -15.9863)
  line L1617 (55.9203, -15.9863) -> (56.1584, -15.9863)
  line L1618 (56.1584, -15.9863) -> (56.3489, -16.034)
  line L1619 (56.3489, -16.034) -> (56.4441, -16.0816)
  line L1620 (56.4441, -16.0816) -> (56.4917, -16.1292)
  line L1621 (56.4917, -16.1292) -> (56.5393, -16.2244)
  line L1622 (56.5393, -16.2244) -> (56.5393, -16.3197)
  line L1623 (56.5393, -16.3197) -> (56.4917, -16.4149)
  line L1624 (56.4917, -16.4149) -> (56.4441, -16.4625)
  line L1625 (56.4441, -16.4625) -> (56.3489, -16.5102)
  line L1626 (56.3489, -16.5102) -> (56.1584, -16.5578)
  line L1627 (56.1584, -16.5578) -> (55.9203, -16.5578)
  line L1628 (55.9203, -16.5578) -> (55.7298, -16.5102)
  line L1629 (55.7298, -16.5102) -> (55.6346, -16.4625)
  line L1630 (55.6346, -16.4625) -> (55.587, -16.4149)
  line L1631 (55.587, -16.4149) -> (55.5393, -16.3197)
  line L1632 (55.8727, -15.1292) -> (56.5393, -15.1292)
  line L1633 (55.4917, -15.3673) -> (56.206, -15.6054)
  line L1634 (56.206, -15.6054) -> (56.206, -14.9863)
  line L1635 (19.4445, -14.4808) -> (19.4445, -12.5008)
  line L1636 (19.4445, -14.4808) -> (4.7245, -14.4808)
  line L1637 (19.4445, -8.8008) -> (19.4445, -0.2607)
  line L1638 (19.4445, -0.2607) -> (4.7245, -0.2607)
  line L1639 (16.0845, -15.3607) -> (15.5845, -14.8607)
  line L1640 (15.5845, -14.8607) -> (15.0845, -15.3607)
  line L1641 (15.0845, -15.3607) -> (16.0845, -15.3607)
  line L1642 (4.7245, -12.5008) -> (4.7245, -14.4808)
  line L1643 (4.7245, -8.8008) -> (4.7245, -0.2607)
  line L1644 (3.8845, -27.616) -> (3.8845, -34.016)
  line L1645 (3.8845, -34.016) -> (6.2845, -34.016)
  line L1646 (4.1345, -26.716) -> (4.1345, -26.516)
  line L1647 (4.7345, -27.616) -> (4.1345, -26.716)
  line L1648 (5.4345, -27.616) -> (6.0345, -26.716)
  line L1649 (6.0345, -26.716) -> (6.0345, -26.516)
  line L1650 (6.2845, -27.616) -> (3.8845, -27.616)
  line L1651 (6.2845, -34.016) -> (6.2845, -27.616)
  circle A0 centre (56.5345, -26.9982) radius 6.1
  line L1652 (11.4445, -17.8682) -> (11.4445, -28.1482)
  line L1653 (11.4445, -28.1482) -> (16.7445, -28.1482)
  line L1654 (13.0945, -17.8682) -> (11.4445, -17.8682)
  line L1655 (16.7445, -17.8682) -> (15.0945, -17.8682)
  line L1656 (16.7445, -28.1482) -> (16.7445, -17.8682)
  arc A1 (13.0945, -17.8682) -> (15.0945, -17.8682) centre (14.0945, -17.8682) cw
  line L1657 (16.4845, -38.8432) -> (17.8145, -38.8432)
  line L1658 (16.4845, -40.1732) -> (16.4845, -38.8432)
  line L1659 (16.4845, -41.4432) -> (16.4845, -51.6632)
  line L1660 (16.4845, -41.4432) -> (19.1445, -41.4432)
  line L1661 (16.4845, -51.6632) -> (19.1445, -51.6632)
  line L1662 (19.1445, -41.4432) -> (19.1445, -51.6632)
  line L1663 (24.5845, -0.4982) -> (24.5845, -0.7982)
  line L1664 (24.5845, -0.4982) -> (45.5845, -0.4982)
  line L1665 (24.5845, -2.8982) -> (24.5845, -3.2982)
  line L1666 (24.5845, -3.1652) -> (27.5915, -3.1652)
  line L1667 (24.5845, -5.4982) -> (24.5845, -5.8983)
  line L1668 (24.5845, -7.9982) -> (24.5845, -8.3983)
  line L1669 (24.5845, -10.5983) -> (24.5845, -10.9982)
  line L1670 (24.5845, -13.0983) -> (24.5845, -13.4982)
  line L1671 (24.5845, -15.5983) -> (24.5845, -15.9982)
  line L1672 (24.5845, -18.1982) -> (24.5845, -18.5983)
  line L1673 (24.5845, -20.6982) -> (24.5845, -21.0983)
  line L1674 (24.5845, -23.2982) -> (24.5845, -23.6983)
  line L1675 (24.5845, -25.7982) -> (24.5845, -26.1983)
  line L1676 (24.5845, -28.2982) -> (24.5845, -28.6983)
  line L1677 (24.5845, -30.8982) -> (24.5845, -31.2982)
  line L1678 (24.5845, -33.3982) -> (24.5845, -33.7982)
  line L1679 (24.5845, -35.9982) -> (24.5845, -36.3982)
  line L1680 (24.5845, -38.4982) -> (24.5845, -38.8982)
  line L1681 (24.5845, -41.0983) -> (24.5845, -41.4982)
  line L1682 (24.5845, -43.5983) -> (24.5845, -43.9982)
  line L1683 (24.5845, -46.0983) -> (24.5845, -46.4982)
  line L1684 (24.5845, -48.6982) -> (24.5845, -49.0983)
  line L1685 (27.5915, -3.1652) -> (27.5915, -0.4982)
  line L1686 (31.3845, -51.4982) -> (24.5845, -51.4982)
  line L1687 (33.5845, -51.4982) -> (33.9845, -51.4982)
  line L1688 (36.1845, -51.4982) -> (36.5845, -51.4982)
  line L1689 (45.5845, -0.4982) -> (45.5845, -0.7982)
  line L1690 (45.5845, -2.8982) -> (45.5845, -3.2982)
  line L1691 (45.5845, -5.4982) -> (45.5845, -5.8983)
  line L1692 (45.5845, -7.9982) -> (45.5845, -8.3983)
  line L1693 (45.5845, -10.5983) -> (45.5845, -10.9982)
  line L1694 (45.5845, -13.0983) -> (45.5845, -13.4982)
  line L1695 (45.5845, -15.5983) -> (45.5845, -15.9982)
  line L1696 (45.5845, -18.1982) -> (45.5845, -18.5983)
  line L1697 (45.5845, -20.6982) -> (45.5845, -21.0983)
  line L1698 (45.5845, -23.2982) -> (45.5845, -23.6983)
  line L1699 (45.5845, -25.7982) -> (45.5845, -26.1983)
  line L1700 (45.5845, -28.2982) -> (45.5845, -28.6983)
  line L1701 (45.5845, -30.8982) -> (45.5845, -31.2982)
  line L1702 (45.5845, -33.3982) -> (45.5845, -33.7982)
  line L1703 (45.5845, -35.9982) -> (45.5845, -36.3982)
  line L1704 (45.5845, -38.4982) -> (45.5845, -38.8982)
  line L1705 (45.5845, -41.0983) -> (45.5845, -41.4982)
  line L1706 (45.5845, -43.5983) -> (45.5845, -43.9982)
  line L1707 (45.5845, -46.0983) -> (45.5845, -46.4982)
  line L1708 (45.5845, -48.6982) -> (45.5845, -49.0983)
  line L1709 (45.5845, -51.4982) -> (38.7845, -51.4982)
  line L1710 (7.2345, -31.2482) -> (13.2345, -31.2482)
  line L1711 (13.2345, -31.2482) -> (13.2345, -54.7482)
  line L1712 (13.2345, -54.7482) -> (7.2345, -54.7482)
  line L1713 (7.2345, -54.7482) -> (7.2345, -31.2482)
  line L1714 (65.4445, -14.4808) -> (65.4445, -12.5008)
  line L1715 (65.4445, -14.4808) -> (50.7245, -14.4808)
  line L1716 (65.4445, -8.8008) -> (65.4445, -0.2607)
  line L1717 (65.4445, -0.2607) -> (50.7245, -0.2607)
  line L1718 (62.0845, -15.3607) -> (61.5845, -14.8607)
  line L1719 (61.5845, -14.8607) -> (61.0845, -15.3607)
  line L1720 (61.0845, -15.3607) -> (62.0845, -15.3607)
  line L1721 (50.7245, -12.5008) -> (50.7245, -14.4808)
  line L1722 (50.7245, -8.8008) -> (50.7245, -0.2607)
  line L1723 (7.9345, -19.5282) -> (7.9345, -15.9282)
  arc A2 (7.923, -19.5667) -> (3.4845, -17.7282) centre (6.0845, -17.7282) cw
  arc A3 (3.4845, -17.7282) -> (7.923, -15.8898) centre (6.0845, -17.7282) cw
  line L1724 (16.4845, -30.1432) -> (17.8145, -30.1432)
  line L1725 (16.4845, -31.4733) -> (16.4845, -30.1432)
  line L1726 (16.4845, -32.7432) -> (16.4845, -37.8832)
  line L1727 (16.4845, -32.7432) -> (19.1445, -32.7432)
  line L1728 (16.4845, -37.8832) -> (19.1445, -37.8832)
  line L1729 (19.1445, -32.7432) -> (19.1445, -37.8832)
  line L1730 (50.7745, -33.7157) -> (52.1045, -33.7157)
  line L1731 (50.7745, -35.0457) -> (50.7745, -33.7157)
  line L1732 (50.7745, -36.3158) -> (50.7745, -51.6157)
  line L1733 (50.7745, -36.3158) -> (53.4345, -36.3158)
  line L1734 (50.7745, -51.6157) -> (53.4345, -51.6157)
  line L1735 (53.4345, -36.3158) -> (53.4345, -51.6157)
  line L1736 (54.9345, -19.5282) -> (54.9345, -15.9282)
  arc A4 (54.923, -19.5667) -> (50.4845, -17.7282) centre (53.0845, -17.7282) cw
  arc A5 (50.4845, -17.7282) -> (54.923, -15.8898) centre (53.0845, -17.7282) cw
  arc A6 (65.0845, 0.0018) -> (70.0845, -4.9982) centre (65.0845, -4.9982) cw
  circle A7 centre (66.5845, -18.4982) radius 1.75
  arc A8 (0.0845, -4.9982) -> (5.0845, 0.0018) centre (5.0845, -4.9982) cw
  line L1737 (0.0845, -4.9982) -> (0.0845, -50.9982)
  arc A9 (70.0845, -50.9982) -> (65.0845, -55.9982) centre (65.0845, -50.9982) cw
  line L1738 (65.0845, -55.9982) -> (5.0845, -55.9982)
  line L1739 (35.0845, 0.0018) -> (5.0845, 0.0018)
  arc A10 (5.0845, -55.9982) -> (0.0845, -50.9982) centre (5.0845, -50.9982) cw
  line L1740 (35.0845, 0.0018) -> (65.0845, 0.0018)
  circle A11 centre (3.8345, -52.2482) radius 1.75
  circle A12 centre (66.5845, -52.2482) radius 1.75
  line L1741 (70.0845, -4.9982) -> (70.0845, -50.9982)
  circle A13 centre (3.0845, -21.9982) radius 1.75
  line L1742 (53.2845, -25.6983) -> (53.9147, -25.6983) construction
  line L1743 (53.9147, -25.6983) -> (53.9147, -24.365) construction
  line L1744 (53.9147, -24.365) -> (53.2845, -24.365) construction
  line L1745 (53.2845, -24.365) -> (53.2845, -25.6983) construction
  line L1746 (4.7245, -0.2607) -> (19.4445, -0.2607)
  line L1747 (19.4445, -0.2607) -> (19.4445, -14.4808)
  line L1748 (19.4445, -14.4808) -> (4.7245, -14.4808)
  line L1749 (4.7245, -14.4808) -> (4.7245, -0.2607)
  line L1750 (50.7245, -0.2607) -> (65.4445, -0.2607)
  line L1751 (65.4445, -0.2607) -> (65.4445, -14.4808)
  line L1752 (65.4445, -14.4808) -> (50.7245, -14.4808)
  line L1753 (50.7245, -14.4808) -> (50.7245, -0.2607)
  line L1754 (24.5845, -0.4982) -> (45.5845, -0.4982)
  line L1755 (45.5845, -0.4982) -> (45.5845, -51.4982)
  line L1756 (45.5845, -51.4982) -> (24.5845, -51.4982)
  line L1757 (24.5845, -51.4982) -> (24.5845, -0.4982)
  line L1758 (16.4845, -38.8432) -> (19.1445, -38.8432)
  line L1759 (19.1445, -38.8432) -> (19.1445, -51.6632)
  line L1760 (19.1445, -51.6632) -> (16.4845, -51.6632)
  line L1761 (16.4845, -51.6632) -> (16.4845, -38.8432)
  line L1762 (16.4845, -30.1432) -> (19.1445, -30.1432)
  line L1763 (19.1445, -30.1432) -> (19.1445, -37.8832)
  line L1764 (19.1445, -37.8832) -> (16.4845, -37.8832)
  line L1765 (16.4845, -37.8832) -> (16.4845, -30.1432)
  line L1766 (50.7745, -33.7157) -> (53.4345, -33.7157)
  line L1767 (53.4345, -33.7157) -> (53.4345, -51.6157)
  line L1768 (53.4345, -51.6157) -> (50.7745, -51.6157)
  line L1769 (50.7745, -51.6157) -> (50.7745, -33.7157)
  line L1770 (16.4845, -30.1432) -> (19.1445, -32.7432)
  line L1771 (16.4845, -32.7432) -> (19.1445, -30.1432)
  line L1772 (16.4845, -38.8432) -> (19.1445, -41.4432)
  line L1773 (16.4845, -41.4432) -> (19.1445, -38.8432)
  line L1774 (50.7745, -33.7157) -> (53.4345, -36.3158)
  line L1775 (53.4345, -33.7157) -> (50.7745, -36.3158)
  line L1776 (52.4545, -35.3658) -> (51.7545, -35.3658)
  line L1777 (51.7545, -35.3658) -> (51.7545, -34.6658)
  line L1778 (51.7545, -34.6658) -> (52.4545, -34.6658)
  line L1779 (52.4545, -34.6658) -> (52.4545, -35.3658)
  line L1780 (52.4545, -35.3658) -> (51.7545, -34.6658) construction
  line L1781 (51.7545, -35.3658) -> (52.4545, -34.6658) construction
  line L1782 (18.1645, -31.7932) -> (17.4645, -31.7932)
  line L1783 (17.4645, -31.7932) -> (17.4645, -31.0932)
  line L1784 (17.4645, -31.0932) -> (18.1645, -31.0932)
  line L1785 (18.1645, -31.0932) -> (18.1645, -31.7932)
  line L1786 (18.1645, -31.7932) -> (17.4645, -31.0932) construction
  line L1787 (17.4645, -31.7932) -> (18.1645, -31.0932) construction
  line L1788 (18.1645, -40.4932) -> (17.4645, -40.4932)
  line L1789 (17.4645, -40.4932) -> (17.4645, -39.7932)
  line L1790 (17.4645, -39.7932) -> (18.1645, -39.7932)
  line L1791 (18.1645, -39.7932) -> (18.1645, -40.4932)
  line L1792 (18.1645, -40.4932) -> (17.4645, -39.7932) construction
  line L1793 (17.4645, -40.4932) -> (18.1645, -39.7932) construction
  line L1794 (17.4645, -34.3332) -> (17.4645, -33.6332)
  line L1795 (17.4645, -33.6332) -> (18.1645, -33.6332)
  line L1796 (18.1645, -34.3332) -> (17.4645, -34.3332)
  line L1797 (18.1645, -33.6332) -> (18.1645, -34.3332)
  line L1798 (17.4645, -36.8732) -> (17.4645, -36.1732)
  line L1799 (17.4645, -36.1732) -> (18.1645, -36.1732)
  line L1800 (18.1645, -36.8732) -> (17.4645, -36.8732)
  line L1801 (18.1645, -36.1732) -> (18.1645, -36.8732)
  line L1802 (17.4645, -42.3332) -> (18.1645, -42.3332)
  line L1803 (17.4645, -43.0332) -> (17.4645, -42.3332)
  line L1804 (18.1645, -43.0332) -> (17.4645, -43.0332)
  line L1805 (18.1645, -42.3332) -> (18.1645, -43.0332)
  line L1806 (17.4645, -44.8732) -> (18.1645, -44.8732)